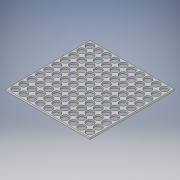
# Autodesk Inventor part: grid2
Saved by Autodesk Inventor 2019 (Build 230136000, 136)
## iProperties
Created: 2019-08-01
Part Number: grid2
Material: Generic
Document SubType Name: Modeling
Designer: assman
Density: 1 g/cm^3
Appearance: Default
Author: assman
## iProperties of the stored document grid2_3DPrint.ipt
Created: 2019-08-01
Part Number: grid2_3DPrint
Material: Generic
Document SubType Name: Modeling
Designer: assman
Density: 1 g/cm^3
Appearance: Default
Author: assman
Autodesk Inventor part; units mm, degrees
ref_plane "YZ Plane" through (0, 0, 0) normal (1, 0, 0) x (0, 1, 0)
ref_plane "XZ Plane" through (0, 0, 0) normal (0, 1, 0) x (-1, 0, 0)
ref_plane "XY Plane" through (0, 0, 0) normal (0, 0, 1) x (1, 0, 0)
sketch "Sketch1" plane through (0, 0, 0) normal (0, 1, 0) x (-1, 0, 0)
  circle A0 centre (19.864, 160.5136) radius 6.1
  line L0 (-59.8031, 200.4081) -> (-59.8031, 68.8047) construction
  line L1 (-59.8031, 68.8047) -> (39.3213, 68.8047) construction
  circle A1 centre (19.864, 146.5136) radius 6.1
  circle A2 centre (19.864, 132.5136) radius 6.1
  circle A3 centre (19.864, 118.5136) radius 6.1
  circle A4 centre (19.864, 104.5136) radius 6.1
  circle A5 centre (19.864, 90.5136) radius 6.1
  circle A6 centre (19.864, 76.5136) radius 6.1
  circle A7 centre (19.864, 62.5136) radius 6.1
  circle A8 centre (19.864, 48.5136) radius 6.1
  circle A9 centre (19.864, 34.5136) radius 6.1
  circle A10 centre (33.864, 160.5136) radius 6.1
  circle A11 centre (33.864, 146.5136) radius 6.1
  circle A12 centre (33.864, 132.5136) radius 6.1
  circle A13 centre (33.864, 118.5136) radius 6.1
  circle A14 centre (33.864, 104.5136) radius 6.1
  circle A15 centre (33.864, 90.5136) radius 6.1
  circle A16 centre (33.864, 76.5136) radius 6.1
  circle A17 centre (33.864, 62.5136) radius 6.1
  circle A18 centre (33.864, 48.5136) radius 6.1
  circle A19 centre (33.864, 34.5136) radius 6.1
  circle A20 centre (47.864, 160.5136) radius 6.1
  circle A21 centre (47.864, 146.5136) radius 6.1
  circle A22 centre (47.864, 132.5136) radius 6.1
  circle A23 centre (47.864, 118.5136) radius 6.1
  circle A24 centre (47.864, 104.5136) radius 6.1
  circle A25 centre (47.864, 90.5136) radius 6.1
  circle A26 centre (47.864, 76.5136) radius 6.1
  circle A27 centre (47.864, 62.5136) radius 6.1
  circle A28 centre (47.864, 48.5136) radius 6.1
  circle A29 centre (47.864, 34.5136) radius 6.1
  circle A30 centre (61.864, 160.5136) radius 6.1
  circle A31 centre (61.864, 146.5136) radius 6.1
  circle A32 centre (61.864, 132.5136) radius 6.1
  circle A33 centre (61.864, 118.5136) radius 6.1
  circle A34 centre (61.864, 104.5136) radius 6.1
  circle A35 centre (61.864, 90.5136) radius 6.1
  circle A36 centre (61.864, 76.5136) radius 6.1
  circle A37 centre (61.864, 62.5136) radius 6.1
  circle A38 centre (61.864, 48.5136) radius 6.1
  circle A39 centre (61.864, 34.5136) radius 6.1
  circle A40 centre (75.864, 160.5136) radius 6.1
  circle A41 centre (75.864, 146.5136) radius 6.1
  circle A42 centre (75.864, 132.5136) radius 6.1
  circle A43 centre (75.864, 118.5136) radius 6.1
  circle A44 centre (75.864, 104.5136) radius 6.1
  circle A45 centre (75.864, 90.5136) radius 6.1
  circle A46 centre (75.864, 76.5136) radius 6.1
  circle A47 centre (75.864, 62.5136) radius 6.1
  circle A48 centre (75.864, 48.5136) radius 6.1
  circle A49 centre (75.864, 34.5136) radius 6.1
  circle A50 centre (89.864, 160.5136) radius 6.1
  circle A51 centre (89.864, 146.5136) radius 6.1
  circle A52 centre (89.864, 132.5136) radius 6.1
  circle A53 centre (89.864, 118.5136) radius 6.1
  circle A54 centre (89.864, 104.5136) radius 6.1
  circle A55 centre (89.864, 90.5136) radius 6.1
  circle A56 centre (89.864, 76.5136) radius 6.1
  circle A57 centre (89.864, 62.5136) radius 6.1
  circle A58 centre (89.864, 48.5136) radius 6.1
  circle A59 centre (89.864, 34.5136) radius 6.1
  circle A60 centre (103.864, 160.5136) radius 6.1
  circle A61 centre (103.864, 146.5136) radius 6.1
  circle A62 centre (103.864, 132.5136) radius 6.1
  circle A63 centre (103.864, 118.5136) radius 6.1
  circle A64 centre (103.864, 104.5136) radius 6.1
  circle A65 centre (103.864, 90.5136) radius 6.1
  circle A66 centre (103.864, 76.5136) radius 6.1
  circle A67 centre (103.864, 62.5136) radius 6.1
  circle A68 centre (103.864, 48.5136) radius 6.1
  circle A69 centre (103.864, 34.5136) radius 6.1
  circle A70 centre (117.864, 160.5136) radius 6.1
  circle A71 centre (117.864, 146.5136) radius 6.1
  circle A72 centre (117.864, 132.5136) radius 6.1
  circle A73 centre (117.864, 118.5136) radius 6.1
  circle A74 centre (117.864, 104.5136) radius 6.1
  circle A75 centre (117.864, 90.5136) radius 6.1
  circle A76 centre (117.864, 76.5136) radius 6.1
  circle A77 centre (117.864, 62.5136) radius 6.1
  circle A78 centre (117.864, 48.5136) radius 6.1
  circle A79 centre (117.864, 34.5136) radius 6.1
  circle A80 centre (131.864, 160.5136) radius 6.1
  circle A81 centre (131.864, 146.5136) radius 6.1
  circle A82 centre (131.864, 132.5136) radius 6.1
  circle A83 centre (131.864, 118.5136) radius 6.1
  circle A84 centre (131.864, 104.5136) radius 6.1
  circle A85 centre (131.864, 90.5136) radius 6.1
  circle A86 centre (131.864, 76.5136) radius 6.1
  circle A87 centre (131.864, 62.5136) radius 6.1
  circle A88 centre (131.864, 48.5136) radius 6.1
  circle A89 centre (131.864, 34.5136) radius 6.1
  circle A90 centre (145.864, 160.5136) radius 6.1
  circle A91 centre (145.864, 146.5136) radius 6.1
  circle A92 centre (145.864, 132.5136) radius 6.1
  circle A93 centre (145.864, 118.5136) radius 6.1
  circle A94 centre (145.864, 104.5136) radius 6.1
  circle A95 centre (145.864, 90.5136) radius 6.1
  circle A96 centre (145.864, 76.5136) radius 6.1
  circle A97 centre (145.864, 62.5136) radius 6.1
  circle A98 centre (145.864, 48.5136) radius 6.1
  circle A99 centre (145.864, 34.5136) radius 6.1
  line L2 (153.964, 26.4136) -> (153.964, 168.6136)
  line L3 (153.964, 168.6136) -> (11.764, 168.6136)
  line L4 (11.764, 168.6136) -> (11.764, 26.4136)
  line L5 (11.764, 26.4136) -> (153.964, 26.4136)
  point P0 (0, 0)
  dimension "d0" = 12.2
  dimension "d3" = 14
  dimension "d6" = 14
  constraints: 100 centre point, 12 end point, 2 parallel, 2 vertical, 1 horizontal, 1 perpendicular, 198 other
  measures "d0" diameter of A0
  measures "d3" distance of A0.centre A1.centre
  measures "d6" distance of A0.centre A10.centre
extrude "Extrusion1" add sketch "Sketch1" along normal blind 3
body "Solid1"
